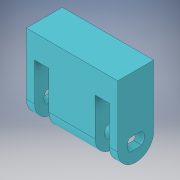
# Autodesk Inventor part: joint1_level
Saved by Autodesk Inventor 2019 (Build 230136000, 136)
## iProperties
Created: 2019-12-26
Part Number: joint1_level
Material: Пластик АБС
Document SubType Name: Modeling
Designer: Петров Иван
Density: 1.06 g/cm^3
Appearance: Серо-синий
Author: Петров Иван
Autodesk Inventor part; units mm, degrees
ref_plane "YZ Plane" through (0, 0, 0) normal (1, 0, 0) x (0, 1, 0)
ref_plane "XZ Plane" through (0, 0, 0) normal (0, 1, 0) x (-1, 0, 0)
ref_plane "XY Plane" through (0, 0, 0) normal (0, 0, 1) x (1, 0, 0)
sketch "Эскиз1" plane through (0, 0, 0) normal (1, 0, 0) x (0, 1, 0)
  line L0 (-6, -6.0208) -> (-6, 6.0208)
  arc A0 (-6, -6.0208) -> (6, -6.0208) centre (0, 0) ccw
  line L1 (6, 6.0208) -> (6, -6.0208)
  arc A1 (6, 6.0208) -> (-6, 6.0208) centre (0, 0) ccw
  circle A2 centre (0, 0) radius 17.5
  line L2 (0, 17.5) -> (60, 17.5)
  line L3 (60, 17.5) -> (60, -17.5)
  line L4 (60, -17.5) -> (0, -17.5)
  line L5 (0, -17.5) -> (0, -8.5)
  line L6 (0, 8.5) -> (0, 17.5)
  dimension "d0" = 35
  dimension "d1" = 60
  constraints: 14 end point, 6 point on circle, 3 parallel, 2 centre point, 1 coincident, 1 horizontal, 1 perpendicular, 1 vertical alignment, 2 other
  measures "d1" distance of L3.end L4.end
extrude "Выдавливание1" add sketch "Эскиз1" along normal blind 45 contours A0 L5 A2 L6 A1 L0 | A0 L1 A1 L6 A2 L5 | A2 L2 L3 L4
sketch "Эскиз2" plane through (45, 0, 0) normal (1, 0, 0) x (0, 0, -1)
  line L0 (17.5, 60) -> (-17.5, 60) projected
  line L1 (17.5, 0) -> (17.5, 60) projected
  line L2 (-17.5, 60) -> (17.5, 60)
  line L3 (17.5, 60) -> (17.5, 37)
  line L4 (17.5, 37) -> (-17.5, 37)
  line L5 (-17.5, 37) -> (-17.5, 60)
  point P0 (0, 0)
  dimension "d4" = 23
  constraints: 8 end point, 2 parallel, 1 horizontal, 1 perpendicular, 1 point on line
  measures "d4" distance of L2.end L3.end
extrude "Выдавливание2" add sketch "Эскиз2" along normal blind 22
ref_plane "РабПлоскость1" through (22.5, 0, 17.5) normal (1, 0, 0) x (0, 0, -1)
mirror "Зеркальное отражение1" about plane through (22.5, 0, 17.5) normal (1, 0, 0) of "Выдавливание2"
sketch "Эскиз3" plane through (45, 0, 0) normal (1, 0, 0) x (0, 0, -1)
  arc A0 (6.0208, -6) -> (6.0208, 6) centre (0, 0) ccw projected
  line L0 (6.0208, -6) -> (-6.0208, -6) projected
  arc A1 (-6.0208, 6) -> (-6.0208, -6) centre (0, 0) ccw projected
  line L1 (6.0208, 6) -> (-6.0208, 6) projected
  line L2 (17.5, 37) -> (-17.5, 37) projected
  line L3 (-17.5, 37) -> (-17.5, 0) projected
  arc A2 (-17.5, 0) -> (17.5, 0) centre (0, 0) ccw projected
  line L4 (17.5, 0) -> (17.5, 37) projected
sketch "Эскиз4" plane through (67, 0, 0) normal (1, 0, 0) x (0, 0, -1)
  arc A0 (6.0208, -6) -> (6.0208, 6) centre (0, 0) ccw
  line L0 (6.0208, -6) -> (-6.0208, -6)
  arc A1 (-6.0208, 6) -> (-6.0208, -6) centre (0, 0) ccw
  line L1 (6.0208, 6) -> (-6.0208, 6)
  line L2 (17.5, 37) -> (-17.5, 37)
  line L3 (-17.5, 37) -> (-17.5, 0)
  arc A2 (-17.5, 0) -> (17.5, 0) centre (0, 0) ccw
  line L4 (17.5, 0) -> (17.5, 37)
  constraints: 10 end point, 6 point on circle, 3 centre point
extrude "Выдавливание3" add sketch "Эскиз4" against normal blind 8
mirror "Зеркальное отражение2" about plane through (22.5, 0, 17.5) normal (1, 0, 0) of "Выдавливание3"
